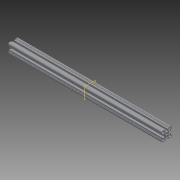
# Autodesk Inventor part: profilato416
Saved by Autodesk Inventor 2014 SP1 (Build 180222100, 222)
## iProperties
Created: 2015-04-08
Part Number: profilato416
Material: Generic
Document SubType Name: Modeling
Designer: Giorgio Nuzzo
Density: 1 g/cm^3
Appearance: Default
Author: Giorgio Nuzzo
Autodesk Inventor part; units mm, degrees
ref_plane "YZ Plane" through (0, 0, 0) normal (1, 0, 0) x (0, 1, 0)
ref_plane "XZ Plane" through (0, 0, 0) normal (0, 1, 0) x (-1, 0, 0)
ref_plane "XY Plane" through (0, 0, 0) normal (0, 0, 1) x (1, 0, 0)
sketch "Sketch1" plane through (0, 0, 0) normal (1, 0, 0) x (0, 1, 0)
  line L0 (0, 25.1698) -> (0, -25.1698) construction
  line L1 (-25.1698, 0) -> (25.1698, 0) construction
  line L2 (-13.75, 13.75) -> (13.75, 13.75) construction
  line L3 (13.75, 13.75) -> (13.75, -13.75) construction
  line L4 (13.75, -13.75) -> (-13.75, -13.75) construction
  line L5 (-13.75, -13.75) -> (-13.75, 13.75) construction
  line L6 (-17.9785, 13.9213) -> (17.1336, 13.9213) construction
  line L7 (17.1336, 13.9213) -> (17.1336, -14.9109) construction
  line L8 (17.1336, -14.9109) -> (-17.9785, -14.9109) construction
  line L9 (-17.9785, -14.9109) -> (-17.9785, 13.9213) construction
  line L10 (5, -5) -> (-5, -5) construction
  line L11 (-5, -5) -> (-5, 5) construction
  line L12 (-5, 5) -> (5, 5) construction
  line L13 (5, 5) -> (5, -5) construction
  line L14 (5, -5) -> (-5, 5) construction
  line L15 (-5, -5) -> (5, 5) construction
  line L16 (-5, 4) -> (-10.25, 4)
  line L17 (-10.25, 4) -> (-10.25, 2.5)
  line L18 (-10.25, 2.5) -> (-11.75, 2.5)
  line L19 (-11.75, 2.5) -> (-11.75, 6)
  line L20 (-11.75, 6) -> (-12.75, 6)
  line L21 (-12.75, 6) -> (-12.75, 8)
  line L22 (-12.75, 8) -> (-13.75, 8)
  line L23 (-13.75, 13.75) -> (0, 0) construction
  line L24 (-4, 5) -> (-4, 10.25)
  line L25 (-4, 10.25) -> (-2.5, 10.25)
  line L26 (-2.5, 10.25) -> (-2.5, 11.75)
  line L27 (-2.5, 11.75) -> (-6, 11.75)
  line L28 (-6, 11.75) -> (-6, 12.75)
  line L29 (-6, 12.75) -> (-8, 12.75)
  line L30 (-8, 12.75) -> (-8, 13.75)
  line L31 (-13.75, 8) -> (-13.75, 10.25)
  line L32 (-8, 13.75) -> (-10.25, 13.75)
  arc A0 (-10.25, 13.75) -> (-13.75, 10.25) centre (-10.25, 10.25) ccw
  line L33 (-5, 5) -> (-10.75, 5)
  line L34 (-10.75, 5) -> (-10.75, 7)
  line L35 (-10.75, 7) -> (-11.75, 7)
  line L36 (-11.75, 7) -> (-11.75, 9)
  line L37 (-11.75, 9) -> (-12.75, 9)
  line L38 (-5, 5) -> (-5, 10.75)
  line L39 (-5, 10.75) -> (-7, 10.75)
  line L40 (-7, 10.75) -> (-7, 11.75)
  line L41 (-7, 11.75) -> (-9, 11.75)
  line L42 (-9, 11.75) -> (-9, 12.75)
  line L43 (-12.75, 9) -> (-12.75, 10.25)
  line L44 (-9, 12.75) -> (-10.25, 12.75)
  arc A1 (-10.25, 12.75) -> (-12.75, 10.25) centre (-10.25, 10.25) ccw
  line L45 (-4, -5) -> (-4, -10.25)
  line L46 (-4, -10.25) -> (-2.5, -10.25)
  line L47 (-2.5, -10.25) -> (-2.5, -11.75)
  line L48 (-2.5, -11.75) -> (-6, -11.75)
  line L49 (-6, -11.75) -> (-6, -12.75)
  line L50 (-6, -12.75) -> (-8, -12.75)
  line L51 (-8, -12.75) -> (-8, -13.75)
  line L52 (-10.25, -4) -> (-10.25, -2.5)
  line L53 (-5, -4) -> (-10.25, -4)
  line L54 (-10.25, -2.5) -> (-11.75, -2.5)
  line L55 (-11.75, -6) -> (-12.75, -6)
  line L56 (-11.75, -2.5) -> (-11.75, -6)
  line L57 (-12.75, -6) -> (-12.75, -8)
  line L58 (-12.75, -8) -> (-13.75, -8)
  line L59 (-8, -13.75) -> (-10.25, -13.75)
  line L60 (-13.75, -8) -> (-13.75, -10.25)
  arc A2 (-13.75, -10.25) -> (-10.25, -13.75) centre (-10.25, -10.25) ccw
  line L61 (-5, -5) -> (-5, -10.75)
  line L62 (-5, -10.75) -> (-7, -10.75)
  line L63 (-7, -10.75) -> (-7, -11.75)
  line L64 (-7, -11.75) -> (-9, -11.75)
  line L65 (-9, -11.75) -> (-9, -12.75)
  line L66 (-11.75, -9) -> (-12.75, -9)
  line L67 (-11.75, -7) -> (-11.75, -9)
  line L68 (-10.75, -7) -> (-11.75, -7)
  line L69 (-10.75, -5) -> (-10.75, -7)
  line L70 (-5, -5) -> (-10.75, -5)
  line L71 (-9, -12.75) -> (-10.25, -12.75)
  line L72 (-12.75, -9) -> (-12.75, -10.25)
  arc A3 (-12.75, -10.25) -> (-10.25, -12.75) centre (-10.25, -10.25) ccw
  line L73 (5, -4) -> (10.25, -4)
  line L74 (10.25, -4) -> (10.25, -2.5)
  line L75 (10.25, -2.5) -> (11.75, -2.5)
  line L76 (11.75, -2.5) -> (11.75, -6)
  line L77 (11.75, -6) -> (12.75, -6)
  line L78 (12.75, -6) -> (12.75, -8)
  line L79 (12.75, -8) -> (13.75, -8)
  line L80 (4, -10.25) -> (2.5, -10.25)
  line L81 (4, -5) -> (4, -10.25)
  line L82 (2.5, -10.25) -> (2.5, -11.75)
  line L83 (6, -11.75) -> (6, -12.75)
  line L84 (2.5, -11.75) -> (6, -11.75)
  line L85 (6, -12.75) -> (8, -12.75)
  line L86 (8, -12.75) -> (8, -13.75)
  line L87 (13.75, -8) -> (13.75, -10.25)
  line L88 (8, -13.75) -> (10.25, -13.75)
  arc A4 (10.25, -13.75) -> (13.75, -10.25) centre (10.25, -10.25) ccw
  line L89 (5, -5) -> (10.75, -5)
  line L90 (10.75, -5) -> (10.75, -7)
  line L91 (10.75, -7) -> (11.75, -7)
  line L92 (11.75, -7) -> (11.75, -9)
  line L93 (11.75, -9) -> (12.75, -9)
  line L94 (9, -11.75) -> (9, -12.75)
  line L95 (7, -11.75) -> (9, -11.75)
  line L96 (7, -10.75) -> (7, -11.75)
  line L97 (5, -10.75) -> (7, -10.75)
  line L98 (5, -5) -> (5, -10.75)
  line L99 (12.75, -9) -> (12.75, -10.25)
  line L100 (9, -12.75) -> (10.25, -12.75)
  arc A5 (10.25, -12.75) -> (12.75, -10.25) centre (10.25, -10.25) ccw
  line L101 (4, 5) -> (4, 10.25)
  line L102 (4, 10.25) -> (2.5, 10.25)
  line L103 (2.5, 10.25) -> (2.5, 11.75)
  line L104 (2.5, 11.75) -> (6, 11.75)
  line L105 (6, 11.75) -> (6, 12.75)
  line L106 (6, 12.75) -> (8, 12.75)
  line L107 (8, 12.75) -> (8, 13.75)
  line L108 (10.25, 4) -> (10.25, 2.5)
  line L109 (5, 4) -> (10.25, 4)
  line L110 (10.25, 2.5) -> (11.75, 2.5)
  line L111 (11.75, 6) -> (12.75, 6)
  line L112 (11.75, 2.5) -> (11.75, 6)
  line L113 (12.75, 6) -> (12.75, 8)
  line L114 (12.75, 8) -> (13.75, 8)
  line L115 (8, 13.75) -> (10.25, 13.75)
  line L116 (13.75, 8) -> (13.75, 10.25)
  arc A6 (13.75, 10.25) -> (10.25, 13.75) centre (10.25, 10.25) ccw
  line L117 (5, 5) -> (5, 10.75)
  line L118 (5, 10.75) -> (7, 10.75)
  line L119 (7, 10.75) -> (7, 11.75)
  line L120 (7, 11.75) -> (9, 11.75)
  line L121 (9, 11.75) -> (9, 12.75)
  line L122 (11.75, 9) -> (12.75, 9)
  line L123 (11.75, 7) -> (11.75, 9)
  line L124 (10.75, 7) -> (11.75, 7)
  line L125 (10.75, 5) -> (10.75, 7)
  line L126 (5, 5) -> (10.75, 5)
  line L127 (9, 12.75) -> (10.25, 12.75)
  line L128 (12.75, 9) -> (12.75, 10.25)
  arc A7 (12.75, 10.25) -> (10.25, 12.75) centre (10.25, 10.25) ccw
  line L129 (0, 0) -> (-2.8284, 2.8284) construction
  line L130 (-2.8284, 2.8284) -> (-3.182, 2.4749)
  line L131 (-3.182, 2.4749) -> (-2.0856, 1.3785)
  line L132 (-2.8284, 2.8284) -> (-2.4749, 3.182)
  line L133 (-2.4749, 3.182) -> (-1.3785, 2.0856)
  line L134 (-3.182, 2.4749) -> (-2.4749, 3.182)
  line L135 (-2.4749, -3.182) -> (-1.3785, -2.0856)
  line L136 (-3.182, -2.4749) -> (-2.0856, -1.3785)
  line L137 (-2.4749, -3.182) -> (-3.182, -2.4749)
  line L138 (3.182, -2.4749) -> (2.0856, -1.3785)
  line L139 (2.4749, -3.182) -> (1.3785, -2.0856)
  line L140 (3.182, -2.4749) -> (2.4749, -3.182)
  line L141 (2.4749, 3.182) -> (1.3785, 2.0856)
  line L142 (3.182, 2.4749) -> (2.0856, 1.3785)
  line L143 (2.4749, 3.182) -> (3.182, 2.4749)
  arc A8 (-2.0856, 1.3785) -> (-2.0856, -1.3785) centre (0, 0) ccw
  arc A9 (-1.3785, -2.0856) -> (1.3785, -2.0856) centre (0, 0) ccw
  arc A10 (2.0856, -1.3785) -> (2.0856, 1.3785) centre (0, 0) ccw
  arc A11 (1.3785, 2.0856) -> (-1.3785, 2.0856) centre (0, 0) ccw
  line L144 (-5, 4) -> (-5, -4)
  line L145 (-4, -5) -> (4, -5)
  line L146 (5, -4) -> (5, 4)
  line L147 (4, 5) -> (-4, 5)
  point P0 (-12.75, 12.75)
  point P1 (-13.75, -13.75)
  point P2 (-13.9213, -17.9785)
  point P3 (-12.75, -12.75)
  point P4 (13.75, -13.75)
  point P5 (17.9785, -13.9213)
  point P6 (12.75, -12.75)
  point P7 (13.75, 13.75)
  point P8 (13.9213, 17.9785)
  point P9 (12.75, 12.75)
  dimension "d0" = 27.5
  dimension "d1" = 27.5
  dimension "d67" = 10
  dimension "d68" = 10
  dimension "d69" = 1
  dimension "d73" = 1.5
  dimension "d74" = 3.5
  dimension "d75" = 1
  dimension "d76" = 2
  dimension "d77" = 1
  dimension "d78" = 1.5
  dimension "d80" = 3.5
  dimension "d81" = 1
  dimension "d82" = 1
  dimension "d83" = 1
  dimension "d84" = 1
  dimension "d85" = 1
  dimension "d88" = 2.5
  dimension "d91" = 360
  dimension "d96" = 4
  dimension "d97" = 0.5
  dimension "d98" = 0.5
  dimension "d102" = 360
  dimension "d120" = 2.5
  constraints: 284 end point, 24 point on circle, 20 point on line, 14 perpendicular, 13 symmetric about line, 12 centre point, 11 parallel, 4 tangent, 2 coincident, 2 horizontal, 2 midpoint, 1 collinear, 298 other
  measures "d0" distance of L2.start L2.end
  measures "d1" distance of L4.end L2.start
  measures "d67" distance of L10.end L11.end
  measures "d68" distance of L11.end L12.end
  measures "d69" distance between parallel lines of L12 L16
  measures "d73" distance of L17.end L18.end
  measures "d74" distance of L18.end L19.end
  measures "d75" distance of L19.end L20.end
  measures "d76" distance of L20.end L21.end
  measures "d77" distance of L21.end L22.end
  measures "d78" distance between parallel lines of L16 L18
  measures "d80" radius of A0
  measures "d81" distance from line of L19 L33.end
  measures "d82" distance of L19.end L35.end
  measures "d83" distance from line of L21.end L36
  measures "d84" distance from line of L21.end L37
  measures "d85" distance from line of L5 L37.end
  measures "d88" radius of A1
  measures "d96" distance of L23.end L129.end
  measures "d97" distance of L129.end L130.end
  measures "d98" distance of L129.end L132.end
  measures "d120" radius of A11
extrude "Extrusion1" add sketch "Sketch1" along normal blind 416
ref_plane "Work Plane1" through (208, 0, 0) normal (1, 0, 0) x (0, 0, -1)
equation "\"d1\" = d0"
equation "\"d68\" = d67"
body "Solid1"
